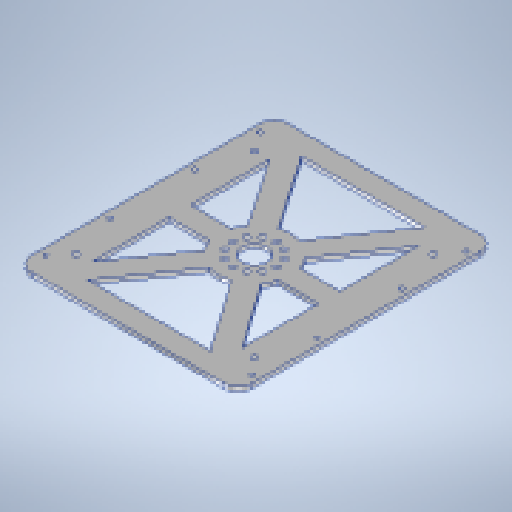
# Autodesk Inventor part: base_plate5
Saved by Autodesk Inventor 2024 (Build 280153000, 153)
## iProperties
Created: 2025-02-14
Part Number: base_plate5
Material: アルミニウム 6061
Document SubType Name: Modeling
Designer: tanoue_kota
Density: 2.7 g/cm^3
Appearance: アルミニウム - フラット
Author: tanoue_kota
Autodesk Inventor part; units mm, degrees
ref_plane "YZ Plane" through (0, 0, 0) normal (1, 0, 0) x (0, 1, 0)
ref_plane "XZ Plane" through (0, 0, 0) normal (0, 1, 0) x (-1, 0, 0)
ref_plane "XY Plane" through (0, 0, 0) normal (0, 0, 1) x (1, 0, 0)
sketch "スケッチ1" plane through (0, 0, 0) normal (0, 1, 0) x (-1, 0, 0)
  line L0 (0, 0) -> (-154, 0)
  line L1 (-154, 0) -> (-154, 178.952)
  line L2 (-154, 178.952) -> (0, 178.952)
  line L3 (0, 178.952) -> (0, 0)
  dimension "d0" = 178.952
  dimension "d1" = 154
  constraints: 8 end point, 2 parallel, 1 horizontal, 1 perpendicular
  measures "d0" distance of L0.end L1.end
  measures "d1" distance of L1.end L2.end
extrude "押し出し1" add sketch "スケッチ1" along normal blind 3
sketch "スケッチ2" plane through (0, 3, 0) normal (0, 1, 0) x (1, 0, 0)
  line L0 (0, 0) -> (0, -178.952) projected
  line L1 (0, -163.952) -> (154, -163.952)
  line L2 (154, -178.952) -> (154, 0) projected
  line L3 (0, -178.952) -> (154, -178.952) projected
  line L4 (0, -118.952) -> (154, -118.952)
  line L5 (0, -15) -> (154, -15)
  line L6 (154, 0) -> (0, 0) projected
  line L7 (0, -60) -> (154, -60)
  line L8 (5, -178.952) -> (5, 0)
  line L9 (149, -178.952) -> (149, -168.1662)
  line L10 (149, -168.1662) -> (149, 0)
  point P0 (5, -163.952)
  point P1 (5, -118.952)
  point P2 (5, -60)
  point P3 (5, -15)
  point P4 (149, -15)
  point P5 (149, -60)
  point P6 (149, -118.952)
  point P7 (149, -163.952)
  dimension "d4" = 15
  dimension "d5" = 45
  dimension "d6" = 15
  dimension "d7" = 45
  dimension "d8" = 5
  dimension "d9" = 5
  constraints: 29 point on line, 14 end point, 5 perpendicular, 1 horizontal
  measures "d4" distance between parallel lines of L3 L1
  measures "d5" distance between parallel lines of L1 L4
  measures "d6" distance between parallel lines of L6 L5
  measures "d7" distance between parallel lines of L5 L7
  measures "d8" distance between parallel lines of L0 L8
  measures "d9" distance between parallel lines of L2 L10
hole "穴1" at (5, 3, 163.952) at (5, 3, 118.952) at (5, 3, 60) at (5, 3, 15) at (149, 3, 15) at (149, 3, 60) at (149, 3, 118.952) at (149, 3, 163.952) direction (0, -1, 0) diameter 3.1 end through all
sketch "スケッチ3" plane through (0, 3, 0) normal (0, 1, 0) x (1, 0, 0)
  circle A0 centre (5, -118.952) radius 1.55 projected
  circle A1 centre (149, -118.952) radius 1.55 projected
  line L0 (5, -118.952) -> (149, -118.952)
  circle A2 centre (149, -60) radius 1.55 projected
  line L1 (149, -118.952) -> (149, -60)
  circle A3 centre (5, -60) radius 1.55 projected
  line L2 (149, -60) -> (5, -60)
  line L3 (5, -60) -> (5, -118.952)
  line L4 (5, -90.476) -> (149, -90.476)
  line L5 (77, -118.952) -> (77, -60)
  circle A4 centre (77, -90.476) radius 15.18
  line L6 (5, -89.476) -> (149, -89.476)
  point P0 (0, 0)
  point P1 (61.82, -90.476)
  point P2 (63.8537, -98.066)
  point P3 (69.41, -103.6223)
  point P4 (77, -105.656)
  point P5 (84.59, -103.6223)
  point P6 (90.1463, -98.066)
  point P7 (92.18, -90.476)
  point P8 (90.1463, -82.886)
  point P9 (84.59, -77.3297)
  point P10 (77, -75.296)
  point P11 (69.41, -77.3297)
  point P12 (63.8537, -82.886)
  dimension "d18" = 30.36
  dimension "d21" = 360
  dimension "d50" = 1
  constraints: 14 end point, 5 midpoint, 4 perpendicular, 4 point on line, 1 horizontal, 1 horizontal alignment, 15 other
  measures "d50" distance between parallel lines of L6 L4
hole "穴2" at (61.82, 3, 90.476) at (63.8537, 3, 98.066) at (69.41, 3, 103.6223) at (77, 3, 105.656) at (84.59, 3, 103.6223) at (90.1463, 3, 98.066) at (92.18, 3, 90.476) at (90.1463, 3, 82.886) at (84.59, 3, 77.3297) at (77, 3, 75.296) at (69.41, 3, 77.3297) at (63.8537, 3, 82.886) direction (0, -1, 0) diameter 4.1 end through all
sketch "スケッチ4" plane through (0, 3, 0) normal (0, 1, 0) x (1, 0, 0)
  circle A0 centre (77, -75.296) radius 2.05 projected
  circle A1 centre (77, -105.656) radius 2.05 projected
  line L0 (77, -75.296) -> (77, -105.656)
  circle A2 centre (77, -90.476) radius 9
  point P0 (0, 0)
  dimension "d30" = 18
  constraints: 2 end point, 1 centre point, 1 midpoint, 1 vertical
  measures "d30" diameter of A2
extrude "押し出し2" cut sketch "スケッチ4" against normal blind 3 contours A2 L0 | L0 A2
sketch "スケッチ5" plane through (0, 3, 0) normal (0, 1, 0) x (1, 0, 0)
  circle A0 centre (77, -90.476) radius 9 projected
  circle A1 centre (77, -90.476) radius 88
  line L0 (77, -90.476) -> (77, -178.476)
  line L1 (77, -90.476) -> (14.7746, -152.7014)
  point P0 (0, 0)
  point P1 (139.2254, -152.7014)
  point P2 (139.2254, -28.2506)
  point P3 (14.7746, -28.2506)
  dimension "d36" = 176
  dimension "d37" = 45
  dimension "d40" = 360
  constraints: 4 end point, 2 coincident, 2 point on circle, 1 centre point, 1 vertical, 5 other
  measures "d36" diameter of A1
  measures "d37" angle of L0 L1
hole "穴3" at (14.7746, 3, 152.7014) at (139.2254, 3, 152.7014) at (139.2254, 3, 28.2506) at (14.7746, 3, 28.2506) direction (0, -1, 0) diameter 4.1 end through all
sketch "スケッチ6" plane through (0, 3, 0) normal (0, 1, 0) x (1, 0, 0)
  line L0 (0, -178.952) -> (154, -178.952) projected
  line L1 (144, -178.952) -> (144, 0)
  line L2 (154, 0) -> (0, 0) projected
  line L3 (154, -178.952) -> (154, 0) projected
  line L4 (10, -178.952) -> (10, 0)
  line L5 (0, 0) -> (0, -178.952) projected
  circle A0 centre (77, -90.476) radius 9 projected
  circle A1 centre (77, -90.476) radius 25
  line L6 (129, -163.952) -> (25, -163.952)
  line L7 (25, -163.952) -> (25, -15)
  line L8 (25, -15) -> (129, -15)
  line L9 (129, -15) -> (129, -163.952)
  line L10 (77, -90.476) -> (25, -163.952)
  line L11 (77, -90.476) -> (129, -15)
  line L12 (77, -90.476) -> (25, -15)
  line L13 (77, -90.476) -> (129, -163.952)
  line L14 (129, -150.969) -> (96.8988, -105.61)
  line L15 (119.8118, -163.952) -> (84.6548, -114.2752)
  line L16 (96.7064, -75.0923) -> (129, -28.2195)
  line L17 (84.3542, -66.5822) -> (119.8923, -15)
  line L18 (69.6458, -66.5822) -> (34.1077, -15)
  line L19 (57.2936, -75.0923) -> (25, -28.2195)
  line L20 (69.3452, -114.2752) -> (34.1882, -163.952)
  line L21 (57.1012, -105.61) -> (25, -150.969)
  line L22 (53.1515, -97.976) -> (25, -97.976)
  line L23 (53.1515, -82.976) -> (25, -82.976)
  line L24 (77, -90.476) -> (10, -90.476)
  line L25 (77, -90.476) -> (77, -163.952)
  line L26 (100.8485, -97.976) -> (129, -97.976)
  line L27 (100.8485, -82.976) -> (129, -82.976)
  point P0 (100.8485, -97.976)
  dimension "d53" = 50
  dimension "d51" = 10
  dimension "d52" = 10
  dimension "d54" = 15
  dimension "d55" = 15
  dimension "d56" = 15
  dimension "d57" = 15
  dimension "d58" = 7.5
  dimension "d59" = 7.5
  dimension "d60" = 7.5
  dimension "d61" = 7.5
  dimension "d62" = 7.5
  dimension "d63" = 7.5
  dimension "d64" = 7.5
  dimension "d65" = 7.5
  dimension "d69" = 7.5
  dimension "d70" = 7.5
  constraints: 48 end point, 15 point on line, 10 parallel, 5 perpendicular, 4 symmetric about line, 1 coincident, 1 horizontal, 1 midpoint, 1 vertical, 12 other
  measures "d51" distance between parallel lines of L3 L1
  measures "d52" distance between parallel lines of L5 L4
  measures "d54" distance between parallel lines of L1 L9
  measures "d55" distance between parallel lines of L0 L6
  measures "d56" distance between parallel lines of L4 L7
  measures "d57" distance between parallel lines of L2 L8
  measures "d58" distance between parallel lines of L13 L14
  measures "d59" distance between parallel lines of L13 L15
  measures "d60" distance between parallel lines of L11 L16
  measures "d61" distance between parallel lines of L11 L17
  measures "d62" distance between parallel lines of L12 L18
  measures "d63" distance between parallel lines of L12 L19
  measures "d64" distance between parallel lines of L20 L10
  measures "d65" distance between parallel lines of L21 L10
  measures "d69" distance between parallel lines of L24 L22
  measures "d70" distance between parallel lines of L24 L23
extrude "押し出し3" cut sketch "スケッチ6" against normal blind 3 contours L22 A1 L21 L7 | L7 L19 A1 L23 | L20 A1 L25 L6 | L8 L17 A1 L18 | L25 A1 L15 L6 | L16 L9 L27 A1 | A1 L26 L9 L14
fillet "フィレット1" radius 10 4 edges at (0, 1.5, 0) (0, 1.5, 178.952) (154, 1.5, 178.952) (154, 1.5, 0)
